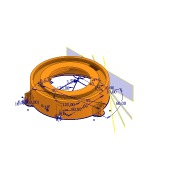
# Autodesk Inventor part: TopPart
Saved by Autodesk Inventor 2020.3 (Build 243373000, 373)
## iProperties
Created: 2021-08-28
Part Number: TopPart
Material: Generic
Document SubType Name: Modeling
Designer: Yusuf
Mass: 36.1951 g
Surface Area: 277.558 cm^2
Volume: 36.1951 cm^3
Density: 1 g/cm^3
Appearance: Orange
Author: Yusuf
Autodesk Inventor part; units mm, degrees
ref_plane "YZ Plane" through (0, 0, 0) normal (1, 0, 0) x (0, 1, 0)
ref_plane "XZ Plane" through (0, 0, 0) normal (0, 1, 0) x (-1, 0, 0)
ref_plane "XY Plane" through (0, 0, 0) normal (0, 0, 1) x (1, 0, 0)
sketch "Sketch1" plane through (0, 0, 0) normal (0, 1, 0) x (-1, 0, 0)
  circle A0 centre (0, 0) radius 47.5
  line L0 (0, 0) -> (23.75, 41.1362)
  line L1 (0, 0) -> (23.75, -41.1362)
  line L2 (0, 0) -> (-47.5, 0)
  circle A1 centre (23.75, 41.1362) radius 8
  circle A2 centre (25.75, 44.6003) radius 1.7
  circle A3 centre (25.75, 44.6003) radius 3.25
  line L3 (23.75, 41.1362) -> (27.75, 48.0644)
  arc A4 (30.4398, 45.5233) -> (30.3168, 36.567) centre (39.3185, 40.9223) ccw
  arc A5 (29.9181, 44.333) -> (29.4758, 46.7233) centre (27.662, 45.1516) ccw
  arc A6 (16.5096, 44.5386) -> (24.2044, 49.1233) centre (15.7805, 54.512) ccw
  arc A7 (25.7257, 48.8884) -> (23.4345, 48.0763) centre (25.2714, 46.5318) ccw
  circle A8 centre (-47.5, 0) radius 8
  arc A9 (-54.6442, 3.6) -> (-46.8263, 7.9716) centre (-55.099, 13.5897) ccw
  circle A10 centre (-51.5, 0) radius 3.25
  circle A11 centre (-51.5, 0) radius 1.7
  line L4 (-47.5, 0) -> (-55.5, 0)
  arc A12 (-53.3526, 3.7433) -> (-55.2014, 2.1651) centre (-52.9334, 1.3802) ccw
  arc A13 (-55.2014, -2.1651) -> (-53.3526, -3.7433) centre (-52.9334, -1.3802) ccw
  arc A14 (-46.8263, -7.9716) -> (-54.6442, -3.6) centre (-55.099, -13.5897) ccw
  circle A15 centre (23.75, -41.1362) radius 8
  arc A16 (24.2044, -49.1233) -> (16.5096, -44.5386) centre (15.7805, -54.512) ccw
  circle A17 centre (25.75, -44.6003) radius 3.25
  circle A18 centre (25.75, -44.6003) radius 1.7
  line L5 (23.75, -41.1362) -> (27.75, -48.0644)
  arc A19 (23.4345, -48.0763) -> (25.7257, -48.8884) centre (25.2714, -46.5318) ccw
  arc A20 (29.4758, -46.7233) -> (29.9181, -44.333) centre (27.662, -45.1516) ccw
  arc A21 (30.3168, -36.567) -> (30.4398, -45.5233) centre (39.3185, -40.9223) ccw
  line L6 (47.2466, -4.9) -> (47.2466, 4.9)
  line L7 (47.2466, 4.9) -> (35.2466, 4.9)
  line L8 (35.2466, 4.9) -> (35.2466, -4.9)
  line L9 (35.2466, -4.9) -> (47.2466, -4.9)
  line L10 (35.2466, -4.9) -> (41.2569, -4.9)
  line L11 (41.2569, -4.9) -> (41.2569, -6.9)
  line L12 (41.2569, -6.9) -> (35.2466, -6.9)
  line L13 (35.2466, -6.9) -> (35.2466, -4.9)
  line L14 (35.2466, 4.9) -> (41.2466, 4.9)
  line L15 (41.2466, 4.9) -> (41.2466, 6.9)
  line L16 (41.2466, 6.9) -> (35.2466, 6.9)
  line L17 (35.2466, 6.9) -> (35.2466, 4.9)
  line L18 (0, 0) -> (-23.75, 41.1362)
  line L19 (-26.3424, 39.5263) -> (-21.0596, 42.5763)
  line L20 (-21.0596, 42.5763) -> (-17.0596, 35.6481)
  line L21 (-17.0596, 35.6481) -> (-22.3424, 32.5981)
  line L22 (-22.3424, 32.5981) -> (-26.3424, 39.5263)
  line L23 (0, 0) -> (-23.75, -41.1362)
  line L24 (0, 0) -> (-30.5324, -36.3871)
  line L25 (0, 0) -> (-16.246, -44.6354)
  line L26 (-24.8744, -25.3659) -> (-20.6611, -28.9012)
  line L27 (-20.6611, -28.9012) -> (-28.3746, -38.0937)
  line L28 (-24.8744, -25.3659) -> (-32.5878, -34.5584)
  line L29 (-20.0917, -29.2999) -> (-15.3286, -32.0499)
  line L30 (-15.3286, -32.0499) -> (-21.3286, -42.4422)
  line L31 (-20.0917, -29.2999) -> (-26.0917, -39.6922)
  line L32 (-14.6986, -32.3437) -> (-9.5303, -34.2248)
  line L33 (-9.5303, -34.2248) -> (-13.6346, -45.5011)
  line L34 (-14.6986, -32.3437) -> (-18.8029, -43.62)
  line L35 (-32.5878, -34.5584) -> (-28.3746, -38.0937)
  line L36 (-26.0917, -39.6922) -> (-21.3286, -42.4422)
  line L37 (-18.8029, -43.62) -> (-13.6346, -45.5011)
  line L38 (20, 30) -> (-20, 30)
  line L39 (-20, 30) -> (-20, -30)
  line L40 (-20, -30) -> (20, -30)
  line L41 (20, -30) -> (20, 30)
  circle A22 centre (17.4, -27.1) radius 1.6
  circle A23 centre (17.4, 27.1) radius 1.6
  circle A24 centre (-17.4, -27.1) radius 1.6
  circle A25 centre (-17.4, 27.1) radius 1.6
  circle A26 centre (0, 38) radius 1.5
  circle A27 centre (0, 38) radius 3
  circle A28 centre (0, 0) radius 45
  line L42 (0, 0) -> (0, -47.5)
  line L43 (-2, -43.4579) -> (2, -43.4579)
  line L44 (2, -43.4579) -> (2, -47.4579)
  line L45 (2, -47.4579) -> (-2, -47.4579)
  line L46 (-2, -47.4579) -> (-2, -43.4579)
  point P0 (-23.75, 0)
  point P1 (16.5096, 44.5386)
  point P2 (25.7257, 48.8884)
  point P3 (-46.8263, 7.9716)
  point P4 (-55.2014, -2.1651)
  point P5 (-46.8263, -7.9716)
  point P6 (29.4758, -46.7233)
  point P7 (30.3168, -36.567)
  point P8 (16.5096, -44.5386)
  point P9 (47.2466, 0)
  point P10 (-19.701, 34.1231)
  point P11 (-23.701, 41.0513)
  point P12 (-22.7677, -27.1335)
  point P13 (-17.7102, -30.6749)
  point P14 (-12.1145, -33.2842)
  point P15 (0, 30)
  point P16 (-20, 0)
  point P17 (-16.3362, 28.2951)
  point P18 (-15.8331, 27.4237)
  point P19 (47.2466, 4.9)
  point P20 (-19.8069, 40.4065)
  point P21 (-25.0896, 37.3565)
  point P22 (44.7324, 4.9)
  point P23 (44.7324, -4.9)
  point P24 (-20, -29.3529)
  point P25 (-18.8791, -30)
  point P26 (0, -43.4579)
  dimension "d0" = 95
  dimension "d1" = 120
  dimension "d2" = 120
  dimension "d3" = 16
  dimension "d4" = 3.4
  dimension "d5" = 6.5
  dimension "d7" = 10
  dimension "d8" = 3.6
  dimension "d9" = 2.4
  dimension "d10" = 1.2
  dimension "d15" = 360
  dimension "d17" = 9.8
  dimension "d18" = 12
  dimension "d19" = 2
  dimension "d20" = 6
  dimension "d21" = 2
  dimension "d23" = 60
  dimension "d24" = 6.1
  dimension "d25" = 8
  dimension "d26" = 6.1
  dimension "d27" = 60
  dimension "d28" = 10
  dimension "d29" = 10
  dimension "LedLength" = 5.5
  dimension "LedWidth" = 12
  dimension "d56" = 40
  dimension "d57" = 60
  dimension "d58" = 3.2
  dimension "d59" = 1.3
  dimension "d60" = 1
  dimension "d61" = 1
  dimension "d62" = 1.3
  dimension "d64" = 3
  dimension "d65" = 8
  dimension "d66" = 6
  dimension "d74" = 90
  dimension "d115" = 4
  dimension "d116" = 4
  constraints: 94 end point, 42 point on circle, 28 centre point, 15 perpendicular, 13 midpoint, 8 parallel, 7 coincident, 7 equal length, 6 symmetric about line, 5 horizontal alignment, 5 point on line, 4 horizontal, 4 vertical alignment, 3 equal radius, 2 vertical, 1 collinear, 1 tangent, 95 other
  measures "d1" angle of L1 L0
  measures "d2" angle of L2 L0
  measures "d3" diameter of A1
  measures "d4" diameter of A2
  measures "d5" diameter of A3
  measures "d7" radius of A4
  measures "d8" distance from line of L3 A1.end
  measures "d9" radius of A5
  measures "d10" vertical distance of A1.end A5.end
  measures "d17" distance of L6.start L6.end
  measures "d18" distance of L6.end L7.end
  measures "d19" distance of L10.end L11.end
  measures "d20" distance of L16.end L15.end
  measures "d21" distance of L15.end L14.end
  measures "d23" angle of L2 L18
  measures "d24" distance of L19.start L19.end
  measures "d25" distance of L19.end L20.end
  measures "d26" distance of L20.end L21.end
  measures "d27" angle of L2 L23
  measures "d28" angle of L24 L23
  measures "d29" angle of L25 L23
  measures "LedLength" distance of L32.start L32.end
  measures "LedWidth" distance of L32.end L33.end
  measures "d56" distance of L40.end L39.end
  measures "d57" distance of L39.end L38.end
  measures "d58" diameter of A22
  measures "d59" distance edge to line of A22 L40
  measures "d60" distance edge to line of A22 L41
  measures "d61" distance edge to line of A25 L39
  measures "d62" distance edge to line of A25 L38
  measures "d64" diameter of A26
  measures "d65" distance from line of L38 A26.centre
  measures "d66" diameter of A27
  measures "d74" diameter of A28
  measures "d115" distance of L44.end L45.end
  measures "d116" distance of L43.end L44.end
ref_plane "Work Plane1" through (32.5878, 0, -34.5584) normal (0.6427876, 0, -0.7660444) x (-0.7660444, 0, -0.6427876)
ref_plane "Work Plane2" through (26.0917, 0, -39.6922) normal (0.5, 0, -0.8660254) x (-0.8660254, 0, -0.5)
ref_plane "Work Plane3" through (18.8029, 0, -43.62) normal (0.3420201, 0, -0.9396926) x (-0.9396926, 0, -0.3420201)
sketch "Sketch2" plane through (32.5878, 0, -34.5584) normal (0.6427876, 0, -0.7660444) x (-0.7660444, 0, -0.6427876)
  line L0 (0, 0) -> (5.5, 0) projected
  circle A0 centre (2.75, 0) radius 2.75
  dimension "d46" = 5.5
  constraints: 1 centre point, 1 coincident
  measures "d46" diameter of A0
sketch "Sketch3" plane through (26.0917, 0, -39.6922) normal (0.5, 0, -0.8660254) x (-0.8660254, 0, -0.5)
  circle A0 centre (2.75, 0) radius 2.75
  dimension "d47" = 5.5
  constraints: 1 centre point, 1 coincident
  measures "d47" diameter of A0
sketch "Sketch4" plane through (18.8029, 0, -43.62) normal (0.3420201, 0, -0.9396926) x (-0.9396926, 0, -0.3420201)
  circle A0 centre (2.75, 0) radius 2.75
  dimension "d48" = 5.5
  constraints: 1 centre point, 1 coincident
  measures "d48" diameter of A0
extrude "Extrusion9" add sketch "Sketch1" along normal blind 26 contours L7 A28 A1 A0 | L6 L9 A28 L7 | A0 A15 A28 L9 | A1 A28 L0 A0 | A0 L1 A28 A15 | L0 A28 A1 A0 | A0 A15 A28 L1 | A1 A28 L20 A0 | A0 L44 A28 A15 | L20 A28 L18 L19 | L45 L42 A28 L44 | A0 L42 L45 | L18 A28 L22 L19 | A0 L45 L42 | L45 L46 A28 L42 | L22 A28 A8 A0 | A0 L33 A28 L46 | A8 A28 L2 A0 | L37 L25 A28 L33 | L2 A28 A8 A0 | L37 L34 A28 L25 | A8 A28 L28 A0 | A0 L30 A28 L34 | A28 L30 L36 L23 | L23 L36 L31 A28 | A28 L27 L35 L24 | L24 L35 L28 A28 | L31 A0 L27 A28
extrude "Extrusion10" cut sketch "Sketch4" against normal up to surface round surface about axis through (0, 0, 0) along (0, 1, 0) radius 45 far side no
extrude "Extrusion11" cut sketch "Sketch3" against normal up to surface round surface about axis through (0, 0, 0) along (0, 1, 0) radius 45 far side no
extrude "Extrusion12" cut sketch "Sketch2" against normal blind 10
extrude "Extrusion13" cut sketch "Sketch1" along normal blind 4.2 contours L20 A28 L18 L19 | L18 A28 L22 L19
extrude "Extrusion14" cut sketch "Sketch1" along normal blind 8.4 contours L6 L9 A28 L7
sketch "Sketch5" plane through (0, 0, 0) normal (1, 0, 0) x (0, 1, 0)
  point P0 (0, 0)
sketch "Sketch6" plane through (0, 26, 0) normal (0, 1, 0) x (1, 0, 0)
  circle A0 centre (0, 0) radius 35
  circle A1 centre (0, 0) radius 42.5
  circle A2 centre (0, 0) radius 25.25
  dimension "d87" = 70
  dimension "d88" = 85
  dimension "d92" = 50.5
  constraints: 3 centre point, 3 coincident
  measures "d87" diameter of A0
  measures "d88" diameter of A1
  measures "d92" diameter of A2
sketch "Sketch7" plane through (0, 0, 0) normal (1, 0, 0) x (0, 1, 0)
  line L0 (26, -42.5) -> (26, 42.5) projected
  line L1 (26, -35) -> (26, 35) projected
  line L2 (26, -47.5) -> (26, -4.9) projected
  line L3 (26, -47.5) -> (26, -44)
  line L4 (0, -39.6922) -> (26, -39.6922) projected
  line L5 (26, -44) -> (22, -44)
  line L6 (22, -44) -> (22, -35.5)
  line L7 (22, -35.5) -> (26, -35.5)
  line L8 (26, -35.5) -> (26, -27.6751)
  line L9 (26, -25.25) -> (26, 25.25) projected
  line L10 (26, -27.6751) -> (26, -25.25)
  line L11 (26, -25.25) -> (22, -25.25)
  line L12 (22, -25.25) -> (22, -23.25)
  line L13 (22, -23.25) -> (20, -23.25)
  line L14 (20, -23.25) -> (20, -47.5)
  line L15 (0, -47.5) -> (26, -47.5) projected
  line L16 (26, -47.5) -> (20, -47.5)
  line L17 (-5.2, 0) -> (31.2, 0) projected
  point P0 (0, 0)
  point P1 (26, -45.5011)
  dimension "d89" = 3.5
  dimension "d90" = 4
  dimension "d91" = 8.5
  dimension "d93" = 2
  dimension "d94" = 2
  dimension "d95" = 4
  constraints: 22 end point, 8 perpendicular, 3 point on line, 1 collinear, 1 horizontal
  measures "d89" distance of L2.start L3.end
  measures "d90" distance of L3.end L5.end
  measures "d91" distance of L5.end L6.end
  measures "d93" distance of L11.end L12.end
  measures "d94" distance of L12.end L13.end
  measures "d95" distance of L9.start L11.end
revolve "Revolution1" add sketch "Sketch7" angle 360 about axis through (0, -10, 0) along (0, 1, 0) contours L2 L15 L14 L4 L6 L5 | L7 L6 L4 L14 L13 L12 L11 L0
extrude "Extrusion15" cut sketch "Sketch1" along normal blind 23.5 contours L38 L41 L40 L1 A22 L0 A23 | L0 A23 L18 A25 L38 | L40 L42 L1 A22 | A23 L0 | L0 A23 | L18 A25 L2 L39 L38 | A22 L1 | L1 A22 | L40 L25 L42 | A25 L18 | L18 A25 | L40 L23 A24 L25 | L24 L39 L2 | L23 A24 L40 L29 L39 L24 | A24 L23 | L23 A24
extrude "Extrusion16" add sketch "Sketch1" along normal blind 12.5 contours A0 L3 A3 A1 A5 A4 | A21 A20 A15 L5 A17 A0 | A0 A6 A7 A1 L3 A3 | L5 A17 A15 A19 A16 A0 | L3 A2 A3 | A3 L3 A2 | L5 A18 A17 | A17 L5 A18 | A0 L4 A10 A8 A12 A9 | A0 A14 A13 A8 L4 A10 | L4 A11 A10 | A10 L4 A11
sketch "Sketch8" plane through (0, 12.5, 0) normal (0, 1, 0) x (1, 0, 0)
  circle A0 centre (-25.75, -44.6003) radius 3.25
  circle A1 centre (-25.75, 44.6003) radius 1.7 projected
  circle A2 centre (-25.75, 44.6003) radius 3
  circle A3 centre (51.5, 0) radius 1.7 projected
  circle A4 centre (51.5, 0) radius 3
  point P0 (0, 0)
  dimension "d101" = 6.5
  dimension "d102" = 6
  dimension "d103" = 6
  constraints: 3 centre point, 3 coincident
  measures "d101" diameter of A0
  measures "d102" diameter of A2
  measures "d103" diameter of A4
extrude "Extrusion17" cut sketch "Sketch8" against normal blind 3
sketch "Sketch9" plane through (0, 20, 0) normal (0, -1, 0) x (1, 0, 0)
  circle A0 centre (0, 0) radius 47.5 projected
  line L0 (-47.2466, -4.9) -> (-47.2466, 4.9) projected
extrude "Extrusion18" add sketch "Sketch9" along normal up to surface (11.6 mm away) contours L0 A0 picked at (-47.3217, 0.5453)
sketch "Sketch10" plane through (0, 22, 0) normal (0, 1, 0) x (1, 0, 0)
  circle A0 centre (0, 0) radius 44 projected
  line L0 (-44, 0) -> (44, 0)
  line L1 (0, -44) -> (0, 44)
  line L2 (0, 0) -> (-7.6405, -43.3315)
  line L3 (0, 0) -> (7.6405, -43.3315)
  line L4 (-6.1743, -35.0161) -> (6.1743, -35.0161)
  circle A1 centre (0, 0) radius 44 projected
  circle A2 centre (0, 0) radius 42.5 projected
  circle A3 centre (0, 0) radius 35.5 projected
  arc A4 (-18.9803, -30) -> (18.9803, -30) centre (0, 0) ccw projected
  line L5 (0, 0) -> (-7.6405, 43.3315)
  line L6 (0, 0) -> (7.6405, 43.3315)
  line L7 (-6.587, 37.3568) -> (6.587, 37.3568)
  point P0 (0, -35.0161)
  point P1 (6.1645, -34.9607)
  point P2 (-6.1645, -34.9607)
  point P3 (0, 37.3568)
  point P4 (-7.6405, 43.3315)
  point P5 (-6.1645, 34.9607)
  point P6 (6.1645, 34.9607)
  point P7 (7.6405, 43.3315)
  dimension "d108" = 20
  dimension "d114" = 20
  constraints: 16 end point, 6 point on circle, 6 point on line, 4 midpoint, 3 horizontal, 1 coincident, 1 vertical, 3 other
  measures "d108" angle of L3 L2
  measures "d114" angle of L6 L5
extrude "Extrusion19" cut sketch "Sketch10" against normal up to surface (2 mm away) contours L6 A2 L1 A0 | L1 A2 L5 A0 | L6 L7 L1 A2 | L1 L7 L5 A2 | L6 A3 L1 L7 | L1 A3 L5 L7
ref_plane "Work Plane4" through (-2, 0, -47.4579) normal (0, 0, -1) x (1, 0, 0)
sketch "Sketch11" plane through (-2, 0, -47.4579) normal (0, 0, -1) x (1, 0, 0)
  circle A0 centre (2, -2.5) radius 2.5
  line L0 (4.5, -2.5) -> (4.5, 0)
  line L1 (14.778, 0) -> (-42.7324, 0) projected
  line L2 (-0.5, -2.5) -> (-0.5, 0)
  line L3 (-14.5096, 0) -> (15.6346, 0) projected
  point P0 (2, 0)
  point P1 (-0.5, 0)
  dimension "d118" = 5
  dimension "d119" = 2.5
  constraints: 4 end point, 2 point on circle, 2 point on line, 2 vertical, 1 centre point, 1 tangent, 1 vertical alignment
  measures "d118" diameter of A0
  measures "d119" distance of point (2, 0) A0.centre
extrude "Extrusion20" cut sketch "Sketch11" along normal mid plane 12
body "Solid2"
